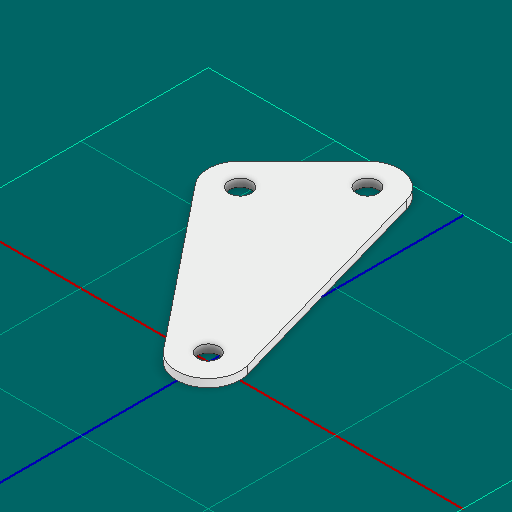
# Autodesk Inventor part: gusset
Saved by Autodesk Inventor 2025 (Build 290162000, 162)
## iProperties
Created: 2024-08-19
Part Number: gusset
Material: Acetal Resin, White
Document SubType Name: Modeling
Designer: averey
Density: 1.425 g/cm^3
Appearance: Smooth - White
Author: averey
Autodesk Inventor part; units mm, degrees
ref_plane "YZ Plane" through (0, 0, 0) normal (1, 0, 0) x (0, 1, 0)
ref_plane "XZ Plane" through (0, 0, 0) normal (0, 1, 0) x (-1, 0, 0)
ref_plane "XY Plane" through (0, 0, 0) normal (0, 0, 1) x (1, 0, 0)
sketch "main" plane through (0, 0, 0) normal (0, 0, 1) x (1, 0, 0)
  circle A0 centre (7.7194, -42.2476) radius 2.1844
  circle A1 centre (20.4194, -29.5476) radius 2.1844
  circle A2 centre (-4.9806, 2.2024) radius 2.0955
  arc A3 (-0.0233, 6.1707) -> (-11.0863, 0.4579) centre (-4.9806, 2.2024) ccw
  arc A4 (1.6137, -43.9921) -> (12.2065, -46.7408) centre (7.7194, -42.2476) ccw
  arc A5 (24.9151, -34.0494) -> (25.3862, -25.5717) centre (20.4194, -29.5476) ccw
  line L0 (12.2065, -46.7408) -> (24.9151, -34.0494)
  line L1 (1.6137, -43.9921) -> (-11.0863, 0.4579)
  line L2 (25.3862, -25.5717) -> (-0.0233, 6.1707)
  point P0 (8.3889, -23.6516)
  dimension "d0" = 12.7
  dimension "d1" = 12.7
  measures "d0" diameter of A3
  measures "d1" diameter of A4
sketch "Sketch1" plane through (0, 0, 0) normal (0, 1, 0) x (-1, 0, 0)
  circle A0 centre (12.7, -44.45) radius 2.1844
  circle A1 centre (25.4, -31.75) radius 2.1844
  circle A2 centre (0, 0) radius 2.0955
  arc A3 (4.9573, 3.9683) -> (-6.1057, -1.7445) centre (0, 0) ccw
  arc A4 (6.5943, -46.1945) -> (17.1871, -48.9432) centre (12.7, -44.45) ccw
  arc A5 (29.8957, -36.2518) -> (30.3668, -27.7741) centre (25.4, -31.75) ccw
  line L0 (17.1871, -48.9432) -> (29.8957, -36.2518)
  line L1 (6.5943, -46.1945) -> (-6.1057, -1.7445)
  line L2 (30.3668, -27.7741) -> (4.9573, 3.9683)
  constraints: 1 other
extrude "Extrusion1" add sketch "Sketch1" along normal blind 1.5875
body "Solid1"
